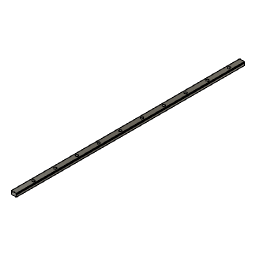
_ProwadnicaLiniowa15_700mm.5dc43066-d862-4f1f-a272-4f7982beec40 (Autodesk Fusion 360 design; units mm, degrees)
Autodesk Fusion 360 part; units mm, degrees
sketch "Sketch1" plane through (0, 0, 0) normal (0, 1, 0) x (1, 0, 0)
  line L0 (0, 0) -> (7.5, 0)
  line L1 (7.5, 0) -> (7.5, -6)
  line L2 (7.5, -6) -> (6.5, -6)
  line L3 (6.5, -6) -> (6.5, -7)
  line L4 (6.5, -7) -> (7.5, -7)
  line L5 (7.5, -7) -> (7.5, -10)
  line L6 (7.5, -10) -> (0, -10)
  line L7 (-7.5, -7) -> (-7.5, -10)
  line L8 (0, 0) -> (-7.5, 0)
  line L9 (-7.5, -6) -> (-6.5, -6)
  line L10 (-7.5, -10) -> (0, -10)
  line L11 (-7.5, 0) -> (-7.5, -6)
  line L12 (-6.5, -6) -> (-6.5, -7)
  line L13 (-6.5, -7) -> (-7.5, -7)
  dimension "d1" = 7.5
  dimension "d2" = 1
  dimension "d3" = 1
  dimension "d4" = 1
  dimension "d5" = 6
  dimension "d6" = 3
  dimension "d7" = 7.5
  constraint coincident L0.start L8.start
  constraint horizontal L0
  constraint perpendicular L0 L1
  constraint perpendicular L1 L2
  constraint perpendicular L2 L3
  constraint perpendicular L3 L4
  constraint perpendicular L4 L5
  constraint perpendicular L5 L6
  measures "d1" distance of L0.start L0.end
  measures "d2" distance of L1.end L2.end
  measures "d3" distance of L2.end L3.end
  measures "d4" distance of L3.end L4.end
  measures "d5" distance of L0.end L1.end
  measures "d6" distance of L4.end L5.end
  measures "d7" distance of L5.end L6.end
extrude "Extrude1" add sketch "Sketch1" along normal blind 700
sketch "Sketch2" plane through (0, 0, 10) normal (0, 0, 1) x (-1, 0, 0)
  line L0 (7.5, 0) -> (-7.5, 0)
  line L1 (-7.5, 0) -> (-7.5, -700)
  line L2 (-7.5, -700) -> (7.5, -700)
  line L3 (7.5, -700) -> (7.5, 0)
  circle A0 centre (0, -60) radius 2.25
  circle A1 centre (0, -126.6667) radius 2.25
  circle A2 centre (0, -193.3333) radius 2.25
  circle A3 centre (0, -260) radius 2.25
  circle A4 centre (0, -326.6667) radius 2.25
  circle A5 centre (0, -393.3333) radius 2.25
  circle A6 centre (0, -460) radius 2.25
  circle A7 centre (0, -526.6667) radius 2.25
  circle A8 centre (0, -593.3333) radius 2.25
  circle A9 centre (0, -660) radius 2.25
  dimension "d10" = 60
  dimension "d12" = 4.5
  measures "d10" distance of origin A0.centre
  measures "d12" diameter of A0
extrude "Extrude2" cut sketch "Sketch2" against normal up to surface (10 mm away) contours A0 | A1 | A2 | A3 | A4 | A5 | A6 | A7 | A8 | A9
sketch "Sketch3" plane through (0, 0, 10) normal (0, 0, 1) x (-1, 0, 0)
  circle A0 centre (0, -526.6667) radius 2.25
  circle A1 centre (0, -260) radius 2.25
  circle A2 centre (0, -60) radius 2.25
  circle A3 centre (0, -326.6667) radius 2.25
  circle A4 centre (0, -593.3333) radius 2.25
  circle A5 centre (0, -460) radius 2.25
  circle A6 centre (0, -193.3333) radius 2.25
  circle A7 centre (0, -126.6667) radius 2.25
  circle A8 centre (0, -393.3333) radius 2.25
  circle A9 centre (0, -660) radius 2.25
  line L0 (7.5, 0) -> (-7.5, 0)
  line L1 (-7.5, 0) -> (-7.5, -700)
  line L2 (-7.5, -700) -> (7.5, -700)
  line L3 (7.5, -700) -> (7.5, 0)
  circle A10 centre (0, -60) radius 3.75
  circle A11 centre (0, -126.6667) radius 3.75
  circle A12 centre (0, -193.3333) radius 3.75
  circle A13 centre (0, -260) radius 3.75
  circle A14 centre (0, -326.6667) radius 3.75
  circle A15 centre (0, -393.3333) radius 3.75
  circle A16 centre (0, -460) radius 3.75
  circle A17 centre (0, -526.6667) radius 3.75
  circle A18 centre (0, -593.3333) radius 3.75
  circle A19 centre (0, -660) radius 3.75
  dimension "d19" = 7.5
  dimension "d22" = 0
  dimension "d23" = -600
  constraint concentric A2 A10
  measures "d19" diameter of A10
extrude "Extrude3" cut sketch "Sketch3" against normal blind 5.3 contours A10 | A11 | A12 | A13 | A14 | A15 | A16 | A17 | A18 | A19
